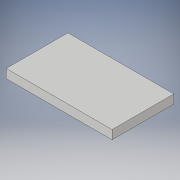
# Autodesk Inventor part: ODS_Enclosure_Top_V1D4
Saved by Autodesk Inventor 2017 (Build 210142000, 142)
## iProperties
Created: 2017-12-29
Part Number: ODS_Enclosure_Top_V1D4
Material: Generic
Document SubType Name: Modeling
Designer: Tripl_000
Density: 1 g/cm^3
Appearance: Default
Author: Tripl_000
Autodesk Inventor part; units mm, degrees
ref_plane "YZ Plane" through (0, 0, 0) normal (1, 0, 0) x (0, 1, 0)
ref_plane "XZ Plane" through (0, 0, 0) normal (0, 1, 0) x (-1, 0, 0)
ref_plane "XY Plane" through (0, 0, 0) normal (0, 0, 1) x (1, 0, 0)
sketch "Sketch1" plane through (0, 0, 0) normal (1, 0, 0) x (0, 1, 0)
  line L0 (1.4605, 13.081) -> (-1.4605, 13.081)
  line L1 (-1.4605, 13.081) -> (-1.4605, -13.081)
  line L2 (-1.4605, -13.081) -> (1.4605, -13.081)
  line L3 (1.4605, -13.081) -> (1.4605, 13.081)
  line L4 (1.4605, 13.081) -> (-1.4605, -13.081) construction
  line L5 (-1.4605, 13.081) -> (1.4605, -13.081) construction
  point P0 (0, 0)
  dimension "d0" = 2.921
  dimension "d1" = 26.162
  constraints: 12 end point, 2 midpoint, 2 parallel, 1 horizontal, 1 perpendicular
  measures "d0" distance between parallel lines of L1 L3
  measures "d1" distance of L2.end L0.start
extrude "Extrusion1" add sketch "Sketch1" along normal blind 120.142
sketch "Sketch2" plane through (0, -1.4605, -13.081) normal (0, -1, 0) x (1, 0, 0)
  line L0 (0, 26.162) -> (120.142, 26.162) projected
  line L1 (75.311, 26.162) -> (44.831, 26.162)
  line L2 (44.831, 26.162) -> (44.831, 19.5072)
  line L3 (44.831, 19.5072) -> (75.311, 19.5072)
  line L4 (75.311, 19.5072) -> (75.311, 26.162)
  line L5 (-38.891, 13.081) -> (135.1376, 13.081)
  line L6 (0, 26.162) -> (0, 0) projected
  line L7 (44.831, 0) -> (44.831, 6.6548)
  line L8 (44.831, 6.6548) -> (75.311, 6.6548)
  line L9 (75.311, 6.6548) -> (75.311, 0)
  line L10 (75.311, 0) -> (44.831, 0)
  line L11 (0, 0) -> (120.142, 0) projected
  point P0 (0, 13.081)
  dimension "d4" = 44.831
  dimension "d5" = 30.48
  dimension "d6" = 6.6548
  constraints: 18 end point, 4 symmetric about line, 2 horizontal, 2 parallel, 1 collinear, 1 perpendicular, 1 point on line
  measures "d4" distance between parallel lines of L6 L2
  measures "d5" distance between parallel lines of L2 L4
  measures "d6" distance between parallel lines of L3 L0
extrude "Extrusion2" cut sketch "Sketch2" against normal through all
sketch "Sketch3" plane through (0, -1.4605, -13.081) normal (0, -1, 0) x (1, 0, 0)
  line L0 (75.311, 19.5072) -> (44.831, 19.5072) projected
  line L1 (75.311, 6.6548) -> (75.311, 0) projected
  line L2 (44.831, 19.5072) -> (75.311, 19.5072)
  line L3 (75.311, 19.5072) -> (75.311, 6.6548)
  line L4 (75.311, 6.6548) -> (44.831, 6.6548)
  line L5 (44.831, 6.6548) -> (44.831, 19.5072)
  point P0 (0, 13.081)
  constraints: 8 end point, 2 parallel, 1 horizontal, 1 perpendicular
extrude "Extrusion3" add sketch "Sketch3" along normal blind 6.35
sketch "Sketch4" plane through (0, 0, 0) normal (-1, 0, 0) x (0, 0, 1)
  line L0 (-13.081, -1.4605) -> (-13.081, 1.4605) projected
  line L1 (13.081, 1.4605) -> (13.081, -1.4605) projected
  line L2 (-44.45, 14.1605) -> (44.45, 14.1605)
  line L3 (-44.45, 14.1605) -> (-44.45, 1.4605)
  line L4 (44.45, 14.1605) -> (44.45, 1.4605)
  line L5 (-44.45, 1.4605) -> (44.45, 1.4605)
  point P0 (0, 0)
  constraints: 8 end point, 2 horizontal, 1 vertical
extrude "Extrusion4" add sketch "Sketch4" against normal up to surface (120.142 mm away)
sketch "Sketch5" plane through (120.142, 0, 0) normal (1, 0, 0) x (0, 0, -1)
  line L0 (44.45, 14.1605) -> (44.45, 1.4605) projected
  line L1 (44.45, 14.1605) -> (-44.45, 14.1605)
  line L2 (-44.45, 14.1605) -> (-44.45, 1.4605)
  line L3 (-44.45, 1.4605) -> (44.45, 1.4605)
  line L4 (44.45, 1.4605) -> (44.45, 14.1605)
  point P0 (0, 0)
  constraints: 8 end point, 2 parallel, 1 horizontal, 1 perpendicular
ref_plane "Work Plane1" through (60.071, 0, 0) normal (1, 0, 0) x (0, 0, -1)
extrude "Extrusion5" add sketch "Sketch5" along normal blind 16.129
mirror "Mirror1" about plane through (60.071, 0, 0) normal (1, 0, 0) of "Extrusion5"
sketch "Sketch6" plane through (136.271, 1.4605, -44.45) normal (0, -1, 0) x (1, 0, 0)
  line L0 (-4.699, 46.99) -> (-9.779, 46.99)
  line L1 (-9.779, 46.99) -> (-9.779, 41.91)
  line L2 (-9.779, 41.91) -> (-4.699, 41.91)
  line L3 (-4.699, 41.91) -> (-4.699, 46.99)
  line L4 (-4.699, 46.99) -> (-9.779, 41.91) construction
  line L5 (-9.779, 46.99) -> (-4.699, 41.91) construction
  line L6 (0, 0) -> (0, 88.9) projected
  line L7 (0, 0) -> (-152.4, 0) projected
  point P0 (-136.271, 44.45)
  point P1 (-7.239, 44.45)
  dimension "d22" = 4.699
  dimension "d23" = 5.08
  dimension "d24" = 5.08
  dimension "d25" = 41.91
  constraints: 12 end point, 2 midpoint, 2 parallel, 1 horizontal, 1 perpendicular
  measures "d22" distance between parallel lines of L6 L3
  measures "d23" distance of L2.end L0.start
  measures "d24" distance of L0.start L0.end
  measures "d25" distance between parallel lines of L7 L2
extrude "Extrusion6" cut sketch "Sketch6" against normal blind 8.89
sketch "Sketch7" plane through (-16.129, 1.4605, -44.45) normal (-1, 0, 0) x (0, 0, 1)
  line L0 (41.91, 8.89) -> (46.99, 8.89)
  line L1 (46.99, 8.89) -> (46.99, 3.81)
  line L2 (46.99, 3.81) -> (41.91, 3.81)
  line L3 (41.91, 3.81) -> (41.91, 8.89)
  line L4 (41.91, 8.89) -> (46.99, 3.81) construction
  line L5 (46.99, 8.89) -> (41.91, 3.81) construction
  line L6 (88.9, 0) -> (0, 0) projected
  line L7 (88.9, 12.7) -> (88.9, 0) projected
  point P0 (44.45, -1.4605)
  point P1 (44.45, 6.35)
  dimension "d28" = 5.08
  dimension "d29" = 5.08
  dimension "d30" = 3.81
  dimension "d31" = 41.91
  constraints: 12 end point, 2 midpoint, 2 parallel, 1 horizontal, 1 perpendicular
  measures "d28" distance of L0.end L1.end
  measures "d29" distance of L0.start L0.end
  measures "d30" distance between parallel lines of L6 L2
  measures "d31" distance between parallel lines of L7 L1
extrude "Extrusion7" cut sketch "Sketch7" against normal up to surface (142.621 mm away)
fillet "Fillet1" radius 3.175 2 edges at (126.492, 5.2705, 0) (131.572, 10.3505, 0)
body "Solid1"
